Autodesk Inventor part; units mm, degrees
(part 2 of 2)
sketch "Skizze13" plane through (0, 0, 0) normal (0, 0, -1) x (-1, 0, 0)
  line L0 (25.1501, -91.41) -> (-3.8499, -91.41) projected
  line L1 (-3.8499, -91.41) -> (-3.8499, -84.41) projected
  line L2 (-3.8499, -84.41) -> (25.1501, -84.41) projected
  line L3 (25.1501, -84.41) -> (25.1501, -91.41) projected
  circle A0 centre (-15, -87.35) radius 1.4 projected
  circle A1 centre (43, -87.35) radius 1.4 projected
  circle A2 centre (43, -38.35) radius 1.4 projected
  circle A3 centre (-15, -38.35) radius 1.4 projected
  line L4 (-21.6433, 21.65) -> (-21.6433, -21.65) projected
  line L5 (21.65, 21.65) -> (-21.6433, 21.65) projected
  line L6 (21.65, -21.65) -> (21.65, 21.65) projected
  line L7 (-21.6433, -21.65) -> (21.65, -21.65) projected
  circle A4 centre (-23.5, 23.5) radius 1.4 projected
  circle A5 centre (-23.5, -23.5) radius 1.4 projected
  circle A6 centre (23.5, 23.5) radius 1.4 projected
  circle A7 centre (23.5, -23.5) radius 1.4 projected
  circle A8 centre (34.65, 27.15) radius 1.6 projected
  circle A9 centre (35.65, 4.15) radius 1.55 projected
  circle A10 centre (56.65, 27.15) radius 1.6 projected
  circle A11 centre (55.65, 4.15) radius 1.55 projected
  line L8 (-28.5, 27.15) -> (-24.5, 31.15) projected
  line L9 (-28.5, -96.85) -> (-28.5, 27.15) projected
  line L10 (-24.5, -100.85) -> (-28.5, -96.85) projected
  line L11 (62.5, -100.85) -> (-24.5, -100.85) projected
  line L12 (66.5, -96.85) -> (62.5, -100.85) projected
  line L13 (66.5, 2.9) -> (66.5, -96.85) projected
  arc A12 (66.5, 5.4) -> (66.5, 2.9) centre (63.5, 4.15) ccw projected
  line L14 (66.5, 25.9) -> (66.5, 5.4) projected
  arc A13 (63.259, 30.391) -> (66.5, 25.9) centre (63.5, 27.15) ccw projected
  line L15 (62.5, 31.15) -> (63.259, 30.391) projected
  line L16 (-24.5, 31.15) -> (62.5, 31.15) projected
  circle A14 centre (-18.5, -90.85) radius 3.25 projected
  circle A15 centre (-18.5, -34.85) radius 3.25 projected
  circle A16 centre (-14.0855, -43.0199) radius 3.25 projected
  circle A17 centre (-14.0855, -77.1359) radius 3.25 projected
  circle A18 centre (61.2633, -96.1146) radius 3.25 projected
  line L17 (10.0034, 17.15) -> (-9.9966, 17.15)
  line L18 (-9.9966, 17.15) -> (-9.9966, 26.15)
  line L19 (-9.9966, 26.15) -> (10.0034, 26.15)
  line L20 (10.0034, 26.15) -> (10.0034, 17.15)
  line L21 (10.0034, 17.15) -> (-9.9966, 26.15) construction
  line L22 (-9.9966, 17.15) -> (10.0034, 26.15) construction
  point P0 (0, 0)
  point P1 (0.0034, 21.65)
  dimension "d80" = 20
  dimension "d81" = 9
  constraints: 12 end point, 3 midpoint, 2 parallel, 1 horizontal, 1 perpendicular
  measures "d80" distance of L18.end L19.end
  measures "d81" distance of L17.end L18.end
extrude "Extrusion7" cut sketch "Skizze13" against normal blind 10 contours L18 L19 L20 L5 | L5 L20 L17 L18
